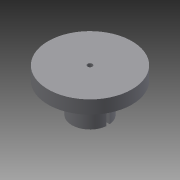
# Autodesk Inventor part: turntable
Saved by Autodesk Inventor 2015 SP2 (Build 190223200, 223)
## iProperties
Created: 2015-05-25
Part Number: turntable
Material: Generic
Document SubType Name: Modeling
Designer: caleb
Density: 1 g/cm^3
Appearance: Default
Author: caleb
Autodesk Inventor part; units mm, degrees
ref_plane "YZ Plane" through (0, 0, 0) normal (1, 0, 0) x (0, 1, 0)
ref_plane "XZ Plane" through (0, 0, 0) normal (0, 1, 0) x (-1, 0, 0)
ref_plane "XY Plane" through (0, 0, 0) normal (0, 0, 1) x (1, 0, 0)
sketch "Sketch1" plane through (0, 0, 0) normal (0, 0, 1) x (1, 0, 0)
  circle A0 centre (0, 0) radius 2.5
  circle A1 centre (0, 0) radius 5.5
  dimension "d0" = 5
  dimension "d1" = 3
  constraints: 2 centre point, 2 coincident
  measures "d0" diameter of A0
  measures "d1" radial gap between concentric circles of A0 A1
extrude "Extrusion1" add sketch "Sketch1" along normal blind 10
sketch "Sketch2" plane through (0, 0, 0) normal (0, 0, -1) x (-1, 0, 0)
  circle A0 centre (0, 0) radius 2.5 construction
  circle A1 centre (0, 0) radius 5.5 construction
  line L0 (-2, 1.5) -> (2, 1.5)
  circle A2 centre (0, 0) radius 2.5 construction
  line L1 (-2, -1.5) -> (2, -1.5)
  arc A3 (-2, 1.5) -> (-2, -1.5) centre (0, 0) ccw
  arc A4 (2, 1.5) -> (-2, 1.5) centre (0, 0) ccw
  arc A5 (2, -1.5) -> (2, 1.5) centre (0, 0) ccw
  arc A6 (-2, -1.5) -> (2, -1.5) centre (0, 0) ccw
  dimension "d4" = 3
  constraints: 15 point on circle, 4 centre point, 4 end point, 2 horizontal, 1 coincident, 1 concentric, 1 parallel
  measures "d4" distance between parallel lines of L0 L1
extrude "Extrusion2" add sketch "Sketch2" against normal blind 10 contours A4 L0 | L1 A6
sketch "Sketch3" plane through (0, 0, 0) normal (1, 0, 0) x (0, 1, 0)
  line L0 (-1.5, 0) -> (1.5, 0) construction
  line L1 (1.5, 0) -> (-1.5, 0) construction
  line L2 (-5.5, 0) -> (5.5, 0) construction
  line L3 (1.5, 10) -> (-1.5, 10) construction
  line L4 (-1.5, 10) -> (1.5, 10) construction
  line L5 (5.5, 10) -> (-5.5, 10) construction
  line L6 (-0.5, 8) -> (0.5, 8)
  line L7 (0.5, 8) -> (0.5, 0)
  line L8 (0.5, 0) -> (-0.5, 0)
  line L9 (-0.5, 0) -> (-0.5, 8)
  point P0 (0, 0)
  point P1 (0, 10)
  point P2 (0, 8)
  dimension "d7" = 8
  dimension "d8" = 1
  constraints: 8 end point, 2 midpoint, 2 parallel, 1 horizontal, 1 perpendicular, 1 point on line, 1 vertical alignment
  measures "d7" distance of L6.end L7.end
  measures "d8" distance between parallel lines of L9 L7
extrude "Extrusion3" cut sketch "Sketch3" along normal through all both and the other way through all
sketch "Sketch4" plane through (0, 0, 10) normal (0, 0, 1) x (1, 0, 0)
  arc A0 (2, -1.5) -> (2, 1.5) centre (0, 0) ccw projected
  line L0 (2, -1.5) -> (-2, -1.5) projected
  arc A1 (-2, 1.5) -> (-2, -1.5) centre (0, 0) ccw projected
  line L1 (-2, 1.5) -> (2, 1.5) projected
  circle A2 centre (0, 0) radius 5.5 projected
extrude "Extrusion4" add sketch "Sketch4" against normal blind 2 contours L0 A1 L1 A0
sketch "Sketch5" plane through (0, 0, 10) normal (0, 0, 1) x (1, 0, 0)
  circle A0 centre (0, 0) radius 5.5 projected
  circle A1 centre (0, 0) radius 12.7
  dimension "d13" = 25.4
  constraints: 1 centre point, 1 coincident
  measures "d13" diameter of A1
extrude "Extrusion5" add sketch "Sketch5" against normal blind 2
sketch "Sketch6" plane through (0, 0, 0) normal (0, 0, -1) x (-1, 0, 0)
  line L0 (5.4772, -0.5) -> (2.4495, -0.5) projected
  arc A0 (2, -1.5) -> (2.4495, -0.5) centre (0, 0) ccw projected
  line L1 (2, -1.5) -> (-2, -1.5) projected
  arc A1 (-2.4495, -0.5) -> (-2, -1.5) centre (0, 0) ccw projected
  line L2 (-2.4495, -0.5) -> (-5.4772, -0.5) projected
  arc A2 (-5.4772, -0.5) -> (5.4772, -0.5) centre (0, 0) ccw projected
  line L3 (2.4495, 0.5) -> (5.4772, 0.5) projected
  arc A3 (5.4772, 0.5) -> (-5.4772, 0.5) centre (0, 0) ccw projected
  line L4 (-5.4772, 0.5) -> (-2.4495, 0.5) projected
  arc A4 (-2, 1.5) -> (-2.4495, 0.5) centre (0, 0) ccw projected
  line L5 (-2, 1.5) -> (2, 1.5) projected
  arc A5 (2.4495, 0.5) -> (2, 1.5) centre (0, 0) ccw projected
  circle A6 centre (0, 0) radius 2.5
  constraints: 1 centre point, 1 coincident, 1 concentric
extrude "Extrusion6" add sketch "Sketch6" along normal blind 1 contours A2 L2 A1 A6 A0 L0 | A6 L1 | A5 A6 A4 L4 A3 L3 | L5 A6
extrude "Extrusion7" cut sketch "Sketch6" along normal through all contours A0 L1 A1 A6 A4 L5 A5 | A6 L1 | L5 A6
sketch "Sketch7" plane through (0, 0, 10) normal (0, 0, 1) x (1, 0, 0)
  circle A0 centre (0, 0) radius 0.75
  dimension "d20" = 1.5
  constraints: 1 centre point, 1 coincident
  measures "d20" diameter of A0
extrude "Extrusion8" cut sketch "Sketch7" against normal through all
sketch "Sketch8" plane through (0, 0, 10) normal (0, 0, 1) x (1, 0, 0)
  circle A0 centre (0, 0) radius 0.75 projected
  circle A1 centre (0, 0) radius 12.7 projected
extrude "Extrusion9" add sketch "Sketch8" along normal blind 2
body "Solid1"
